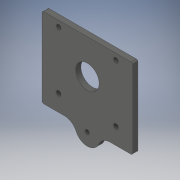
# Autodesk Inventor part: z gearing adapter bottom
Saved by Autodesk Inventor 2019 (Build 230136000, 136)
## iProperties
Created: 2018-07-27
Part Number: z gearing adapter bottom
Material: Generic
Document SubType Name: Modeling
Designer: torba
Density: 1 g/cm^3
Appearance: Gray
Author: torba
Autodesk Inventor part; units mm, degrees
ref_plane "YZ Plane" through (0, 0, 0) normal (1, 0, 0) x (0, 1, 0)
ref_plane "XZ Plane" through (0, 0, 0) normal (0, 1, 0) x (-1, 0, 0)
ref_plane "XY Plane" through (0, 0, 0) normal (0, 0, 1) x (1, 0, 0)
sketch "Sketch1" plane through (0, 0, 0) normal (0, 0, 1) x (1, 0, 0)
  arc A0 (44.2015, -79.5823) -> (38.6015, -79.5823) centre (41.4015, -79.5823) ccw
  arc A1 (38.6015, -85.1823) -> (44.2015, -85.1823) centre (41.4015, -85.1823) ccw
  line L0 (38.6015, -85.1823) -> (38.6015, -79.5823)
  line L1 (44.2015, -79.5823) -> (44.2015, -85.1823)
  arc A2 (39.4335, -50.3778) -> (112.9665, -50.3778) centre (76.2, -50.3778) ccw
  arc A3 (112.9665, -44.7898) -> (39.4335, -44.7898) centre (76.2, -44.7898) ccw
  line L2 (39.4335, -50.3778) -> (39.4335, -44.7898)
  line L3 (112.9665, -44.7898) -> (112.9665, -50.3778)
  line L4 (44.2015, -9.9853) -> (44.2015, -15.5853)
  arc A4 (44.2015, -9.9853) -> (38.6015, -9.9853) centre (41.4015, -9.9853) ccw
  line L5 (38.6015, -15.5853) -> (38.6015, -9.9853)
  arc A5 (38.6015, -15.5853) -> (44.2015, -15.5853) centre (41.4015, -15.5853) ccw
  line L6 (108.1985, -85.1823) -> (108.1985, -79.5823)
  arc A6 (108.1985, -85.1823) -> (113.7985, -85.1823) centre (110.9985, -85.1823) ccw
  line L7 (113.7985, -79.5823) -> (113.7985, -85.1823)
  arc A7 (113.7985, -79.5823) -> (108.1985, -79.5823) centre (110.9985, -79.5823) ccw
  line L8 (108.1985, -15.5853) -> (108.1985, -9.9853)
  arc A8 (113.7985, -9.9853) -> (108.1985, -9.9853) centre (110.9985, -9.9853) ccw
  line L9 (113.7985, -9.9853) -> (113.7985, -15.5853)
  arc A9 (108.1985, -15.5853) -> (113.7985, -15.5853) centre (110.9985, -15.5853) ccw
  circle A10 centre (76.2, -47.5838) radius 1.27
  line L10 (6.35, 0.0014) -> (6.35, -109.7489)
  line L11 (152.4, 0) -> (0, 0)
  line L12 (146.05, 0.0027) -> (146.05, -109.7476)
  line L13 (0, -109.7503) -> (152.4, -109.7503)
  line L14 (21.2, 7.4162) -> (131.2, 7.4162)
  line L15 (131.2, 7.4162) -> (131.2, -102.5838)
  line L16 (131.2, -102.5838) -> (21.2, -102.5838)
  line L17 (21.2, -102.5838) -> (21.2, 7.4162)
  line L18 (21.2, 7.4162) -> (131.2, -102.5838) construction
  line L19 (131.2, 7.4162) -> (21.2, -102.5838) construction
  dimension "d0" = 2.8
  dimension "d1" = 36.7665
  dimension "d2" = 2.54
  dimension "d3" = 90
  dimension "d4" = 90
  dimension "d5" = 90
  dimension "d6" = 90
  dimension "d7" = 109.7503
  dimension "d8" = 32.2515
  dimension "d9" = 33.0835
  dimension "d10" = 101.8485
  dimension "d11" = 139.7
  dimension "d12" = 6.35
  dimension "d13" = 38.6015
  dimension "d14" = 6.35
  dimension "d15" = 0.0027
  dimension "d16" = 37.8515
  dimension "d17" = 109.7476
  dimension "d18" = 9.9853
  dimension "d19" = 69.597
  dimension "d20" = 75.197
  dimension "d21" = 79.5823
  dimension "d22" = 44.7898
  dimension "d23" = 50.3778
  dimension "d24" = 47.5838
  dimension "d25" = 69.85
  dimension "d26" = 9.9853
  dimension "d27" = 79.5823
  dimension "d28" = 0.0014
  dimension "d29" = 109.7489
  dimension "d30" = 146.05
  dimension "d31" = 146.05
  dimension "d32" = 110
  dimension "d33" = 110
  dimension "d34" = 17.4015
  constraints: 40 end point, 24 tangent, 20 point on circle, 11 centre point, 10 parallel, 2 horizontal, 2 midpoint, 1 equal radius, 1 perpendicular, 1 vertical
  measures "d0" radius of A8
  measures "d1" radius of A3
  measures "d2" diameter of A10
  measures "d3" angle of L11 L9
  measures "d4" angle of L11 L8
  measures "d5" angle of L11 L1
  measures "d6" angle of L11 L0
  measures "d7" distance between parallel lines of L11 L13
  measures "d8" distance between parallel lines of L12 L7
  measures "d9" distance between parallel lines of L12 L3
  measures "d10" distance between parallel lines of L12 L4
  measures "d11" distance between parallel lines of L12 L10
  measures "d12" distance from line of L11.start L12
  measures "d13" distance from line of L11.start L9
  measures "d14" distance from line of L13.end L12
  measures "d15" distance from line of L12.start L11
  measures "d16" distance from line of L12.start L8
  measures "d17" distance from line of L12.end L11
  measures "d18" distance from line of L9.start L11
  measures "d19" distance from line of L9.start L1
  measures "d20" distance from line of L9.start L0
  measures "d21" distance from line of L7.start L11
  measures "d22" distance from line of L3.start L11
  measures "d23" distance from line of L3.end L11
  measures "d24" distance from line of A10.centre L11
  measures "d25" distance from line of A10.centre L12
  measures "d26" distance from line of L4.start L11
  measures "d27" distance from line of L1.start L11
  measures "d28" distance from line of L10.start L11
  measures "d29" distance from line of L10.end L11
  measures "d30" distance from line of L11.end L12
  measures "d31" distance from line of L13.start L12
  measures "d32" distance between parallel lines of L15 L17
  measures "d33" distance between parallel lines of L16 L14
  measures "d34" distance from line of L16 A1.centre
extrude "Extrusion1" add sketch "Sketch1" along normal blind 6.35 contours L15 L16 L17 L11 | L11 L17 L14 L15
sketch "Sketch4" plane through (0, 0, 6.35) normal (0, 0, 1) x (1, 0, 0)
  line L0 (112.9665, -44.7898) -> (112.9665, -50.3778) projected
  arc A0 (39.4335, -50.3778) -> (112.9665, -50.3778) centre (76.2, -50.3778) ccw projected
  line L1 (39.4335, -50.3778) -> (39.4335, -44.7898) projected
  arc A1 (112.9665, -44.7898) -> (39.4335, -44.7898) centre (76.2, -44.7898) ccw projected
  arc A2 (38.6015, -15.5853) -> (44.2015, -15.5853) centre (41.4015, -15.5853) ccw projected
  line L2 (38.6015, -15.5853) -> (38.6015, -9.9853) projected
  arc A3 (44.2015, -9.9853) -> (38.6015, -9.9853) centre (41.4015, -9.9853) ccw projected
  line L3 (44.2015, -9.9853) -> (44.2015, -15.5853) projected
  line L4 (44.2015, -79.5823) -> (44.2015, -85.1823) projected
  arc A4 (38.6015, -85.1823) -> (44.2015, -85.1823) centre (41.4015, -85.1823) ccw projected
  line L5 (38.6015, -85.1823) -> (38.6015, -79.5823) projected
  arc A5 (44.2015, -79.5823) -> (38.6015, -79.5823) centre (41.4015, -79.5823) ccw projected
  arc A6 (113.7985, -79.5823) -> (108.1985, -79.5823) centre (110.9985, -79.5823) ccw projected
  line L6 (113.7985, -79.5823) -> (113.7985, -85.1823) projected
  arc A7 (108.1985, -85.1823) -> (113.7985, -85.1823) centre (110.9985, -85.1823) ccw projected
  line L7 (108.1985, -85.1823) -> (108.1985, -79.5823) projected
  arc A8 (113.7985, -9.9853) -> (108.1985, -9.9853) centre (110.9985, -9.9853) ccw projected
  line L8 (113.7985, -9.9853) -> (113.7985, -15.5853) projected
  arc A9 (108.1985, -15.5853) -> (113.7985, -15.5853) centre (110.9985, -15.5853) ccw projected
  line L9 (108.1985, -15.5853) -> (108.1985, -9.9853) projected
  line L10 (21.2, 7.4162) -> (21.2, -102.5838) projected
  line L11 (21.2, -102.5838) -> (131.2, -102.5838) projected
  line L12 (131.2, -102.5838) -> (131.2, 7.4162) projected
  line L13 (76.2, -50.3778) -> (76.2, -44.7898)
  line L14 (76.2, 59.6222) -> (76.2, 65.2102)
  circle A10 centre (76.2, -47.5838) radius 0.5
  circle A11 centre (76.2, 62.4162) radius 0.5
  line L15 (131.2, 7.4162) -> (21.2, 7.4162) projected
  point P0 (0, 0)
  dimension "d72" = 1
  dimension "d73" = 1
  constraints: 4 end point, 2 centre point, 2 midpoint, 2 vertical
  measures "d72" diameter of A10
  measures "d73" diameter of A11
sketch "Sketch11" plane through (0, 0, 6.35) normal (0, 0, 1) x (1, 0, 0)
  line L0 (112.9665, -44.7898) -> (112.9665, -50.3778) projected
  arc A0 (39.4335, -50.3778) -> (112.9665, -50.3778) centre (76.2, -50.3778) ccw projected
  line L1 (39.4335, -50.3778) -> (39.4335, -44.7898) projected
  arc A1 (112.9665, -44.7898) -> (39.4335, -44.7898) centre (76.2, -44.7898) ccw projected
  arc A2 (38.6015, -15.5853) -> (44.2015, -15.5853) centre (41.4015, -15.5853) ccw projected
  line L2 (38.6015, -15.5853) -> (38.6015, -9.9853) projected
  arc A3 (44.2015, -9.9853) -> (38.6015, -9.9853) centre (41.4015, -9.9853) ccw projected
  line L3 (44.2015, -9.9853) -> (44.2015, -15.5853) projected
  line L4 (44.2015, -79.5823) -> (44.2015, -85.1823) projected
  arc A4 (38.6015, -85.1823) -> (44.2015, -85.1823) centre (41.4015, -85.1823) ccw projected
  line L5 (38.6015, -85.1823) -> (38.6015, -79.5823) projected
  arc A5 (44.2015, -79.5823) -> (38.6015, -79.5823) centre (41.4015, -79.5823) ccw projected
  arc A6 (113.7985, -79.5823) -> (108.1985, -79.5823) centre (110.9985, -79.5823) ccw projected
  line L6 (113.7985, -79.5823) -> (113.7985, -85.1823) projected
  arc A7 (108.1985, -85.1823) -> (113.7985, -85.1823) centre (110.9985, -85.1823) ccw projected
  line L7 (108.1985, -85.1823) -> (108.1985, -79.5823) projected
  arc A8 (113.7985, -9.9853) -> (108.1985, -9.9853) centre (110.9985, -9.9853) ccw projected
  line L8 (113.7985, -9.9853) -> (113.7985, -15.5853) projected
  arc A9 (108.1985, -15.5853) -> (113.7985, -15.5853) centre (110.9985, -15.5853) ccw projected
  line L9 (108.1985, -15.5853) -> (108.1985, -9.9853) projected
  line L10 (131.2, 7.4162) -> (21.2, 7.4162) projected
  line L11 (21.2, 7.4162) -> (21.2, -102.5838) projected
  line L12 (21.2, -102.5838) -> (131.2, -102.5838) projected
  line L13 (131.2, -102.5838) -> (131.2, 7.4162) projected
  point P0 (0, 0)
extrude "Extrusion8" add sketch "Sketch11" against normal blind 6.35 contours L0 A0 L1 A1
hole "Hole2" at (76.2, -47.5838, 6.35) direction (0, 0, -1) diameter 28.575 end through all
sketch "Sketch12" plane through (0, 0, 6.35) normal (0, 0, 1) x (1, 0, 0)
  circle A0 centre (76.2, -47.5838) radius 14.2875 projected
  arc A1 (38.6015, -15.5853) -> (44.2015, -15.5853) centre (41.4015, -15.5853) ccw projected
  line L0 (38.6015, -15.5853) -> (38.6015, -9.9853) projected
  arc A2 (44.2015, -9.9853) -> (38.6015, -9.9853) centre (41.4015, -9.9853) ccw projected
  line L1 (44.2015, -9.9853) -> (44.2015, -15.5853) projected
  line L2 (44.2015, -79.5823) -> (44.2015, -85.1823) projected
  arc A3 (38.6015, -85.1823) -> (44.2015, -85.1823) centre (41.4015, -85.1823) ccw projected
  line L3 (38.6015, -85.1823) -> (38.6015, -79.5823) projected
  arc A4 (44.2015, -79.5823) -> (38.6015, -79.5823) centre (41.4015, -79.5823) ccw projected
  arc A5 (113.7985, -79.5823) -> (108.1985, -79.5823) centre (110.9985, -79.5823) ccw projected
  line L4 (113.7985, -79.5823) -> (113.7985, -85.1823) projected
  arc A6 (108.1985, -85.1823) -> (113.7985, -85.1823) centre (110.9985, -85.1823) ccw projected
  line L5 (108.1985, -85.1823) -> (108.1985, -79.5823) projected
  arc A7 (113.7985, -9.9853) -> (108.1985, -9.9853) centre (110.9985, -9.9853) ccw projected
  line L6 (113.7985, -9.9853) -> (113.7985, -15.5853) projected
  arc A8 (108.1985, -15.5853) -> (113.7985, -15.5853) centre (110.9985, -15.5853) ccw projected
  line L7 (108.1985, -15.5853) -> (108.1985, -9.9853) projected
  line L8 (131.2, 7.4162) -> (21.2, 7.4162) projected
  line L9 (21.2, 7.4162) -> (21.2, -102.5838) projected
  line L10 (21.2, -102.5838) -> (131.2, -102.5838) projected
  line L11 (131.2, -102.5838) -> (131.2, 7.4162) projected
  line L12 (21.2, -102.5838) -> (21.2, 7.4162) projected
  line L13 (131.2, 7.4162) -> (131.2, -102.5838) projected
  line L14 (21.2, 7.4162) -> (131.2, 7.4162)
  line L15 (131.2, 7.4162) -> (131.2, 0.8147)
  line L16 (131.2, 0.8147) -> (21.2, 0.8147)
  line L17 (21.2, 0.8147) -> (21.2, 7.4162)
  point P0 (0, 0)
  dimension "d103" = 8
  constraints: 8 end point, 2 parallel, 1 horizontal, 1 perpendicular, 1 point on line
  measures "d103" distance edge to line of A2 L16
extrude "Extrusion9" cut sketch "Sketch12" against normal blind 6.35 contours L11 L16 L9 L8
sketch "Sketch13" plane through (0, 0, 6.35) normal (0, 0, 1) x (1, 0, 0)
  line L0 (131.2, 0.8147) -> (21.2, 0.8147) projected
  line L1 (21.2, 0.8147) -> (21.2, -102.5838) projected
  line L2 (21.2, -102.5838) -> (131.2, -102.5838) projected
  line L3 (131.2, -102.5838) -> (131.2, 0.8147) projected
  arc A0 (113.7985, -9.9853) -> (108.1985, -9.9853) centre (110.9985, -9.9853) ccw projected
  line L4 (113.7985, -9.9853) -> (113.7985, -15.5853) projected
  arc A1 (108.1985, -15.5853) -> (113.7985, -15.5853) centre (110.9985, -15.5853) ccw projected
  line L5 (108.1985, -15.5853) -> (108.1985, -9.9853) projected
  arc A2 (113.7985, -79.5823) -> (108.1985, -79.5823) centre (110.9985, -79.5823) ccw projected
  line L6 (113.7985, -79.5823) -> (113.7985, -85.1823) projected
  arc A3 (108.1985, -85.1823) -> (113.7985, -85.1823) centre (110.9985, -85.1823) ccw projected
  line L7 (108.1985, -85.1823) -> (108.1985, -79.5823) projected
  line L8 (44.2015, -79.5823) -> (44.2015, -85.1823) projected
  arc A4 (38.6015, -85.1823) -> (44.2015, -85.1823) centre (41.4015, -85.1823) ccw projected
  line L9 (38.6015, -85.1823) -> (38.6015, -79.5823) projected
  arc A5 (44.2015, -79.5823) -> (38.6015, -79.5823) centre (41.4015, -79.5823) ccw projected
  arc A6 (38.6015, -15.5853) -> (44.2015, -15.5853) centre (41.4015, -15.5853) ccw projected
  line L10 (38.6015, -15.5853) -> (38.6015, -9.9853) projected
  arc A7 (44.2015, -9.9853) -> (38.6015, -9.9853) centre (41.4015, -9.9853) ccw projected
  line L11 (44.2015, -9.9853) -> (44.2015, -15.5853) projected
  circle A8 centre (76.2, -47.5838) radius 14.2875 projected
  line L12 (41.4015, -85.1823) -> (41.4015, -79.5823)
  line L13 (41.4015, -15.5853) -> (41.4015, -9.9853)
  line L14 (110.9985, -85.1823) -> (110.9985, -79.5823)
  line L15 (41.4015, -85.1823) -> (41.4015, -79.5823) construction
  line L16 (44.2015, -85.1823) -> (44.2015, -79.5823)
  line L17 (38.6015, -79.5823) -> (38.6015, -85.1823)
  arc A9 (38.6015, -85.1823) -> (44.2015, -85.1823) centre (41.4015, -85.1823) ccw
  arc A10 (44.2015, -79.5823) -> (38.6015, -79.5823) centre (41.4015, -79.5823) ccw
  arc A11 (44.2015, -9.9853) -> (38.6015, -9.9853) centre (41.4015, -9.9853) ccw projected
  line L18 (41.4015, -15.5853) -> (41.4015, -9.9853) construction
  line L19 (44.2015, -15.5853) -> (44.2015, -9.9853)
  line L20 (38.6015, -9.9853) -> (38.6015, -15.5853)
  arc A12 (38.6015, -15.5853) -> (44.2015, -15.5853) centre (41.4015, -15.5853) ccw
  arc A13 (44.2015, -9.9853) -> (38.6015, -9.9853) centre (41.4015, -9.9853) ccw
  line L21 (110.9985, -85.1823) -> (110.9985, -79.5823) construction
  line L22 (113.7985, -85.1823) -> (113.7985, -79.5823)
  line L23 (108.1985, -79.5823) -> (108.1985, -85.1823)
  arc A14 (108.1985, -85.1823) -> (113.7985, -85.1823) centre (110.9985, -85.1823) ccw
  arc A15 (113.7985, -79.5823) -> (108.1985, -79.5823) centre (110.9985, -79.5823) ccw
  line L24 (110.9985, -15.5853) -> (110.9985, -9.9853) construction
  line L25 (113.7985, -15.5853) -> (113.7985, -9.9853)
  line L26 (108.1985, -9.9853) -> (108.1985, -15.5853)
  arc A16 (108.1985, -15.5853) -> (113.7985, -15.5853) centre (110.9985, -15.5853) ccw
  arc A17 (113.7985, -9.9853) -> (108.1985, -9.9853) centre (110.9985, -9.9853) ccw
  line L27 (110.9985, -9.9853) -> (110.9985, -15.5853)
  circle A18 centre (110.9985, -12.7853) radius 2.8
  circle A19 centre (41.4015, -12.7853) radius 2.8
  circle A20 centre (41.4015, -82.3823) radius 2.8
  circle A21 centre (110.9985, -82.3823) radius 2.8
  point P0 (0, 0)
  dimension "d108" = 2.8
  dimension "d109" = 2.8
  dimension "d110" = 2.8
  constraints: 40 end point, 21 tangent, 16 point on circle, 12 centre point, 8 equal length, 4 coincident, 4 midpoint, 3 vertical
  measures "d108" radius of A17
  measures "d109" radius of A15
  measures "d110" radius of A10
extrude "Extrusion10" add sketch "Sketch13" against normal blind 6.35 contours L4 A18 L5 A0 | L4 A1 L5 A18 | L6 A21 L7 A2 | L6 A3 L7 A21 | L8 A20 L9 A5 | L8 A4 L9 A20 | L10 A19 L11 A6 | L10 A7 L11 A19
sketch "Sketch17" plane through (0, 0, 6.35) normal (0, 0, 1) x (1, 0, 0)
  circle A0 centre (76.2, -105.7258) radius 4
  circle A1 centre (76.2, -105.7258) radius 2.5
  circle A2 centre (41.4015, -82.3823) radius 2.8
  circle A3 centre (41.4015, -82.3823) radius 2.8 projected
  circle A4 centre (76.2, -105.7258) radius 15
  line L0 (21.2, -102.5838) -> (131.2, -102.5838) projected
  line L1 (131.2, -102.5838) -> (131.2, 0.8147) projected
  line L2 (131.2, 0.8147) -> (21.2, 0.8147) projected
  line L3 (21.2, 0.8147) -> (21.2, -102.5838) projected
  circle A5 centre (110.9985, -12.7853) radius 2.8 projected
  circle A6 centre (110.9985, -82.3823) radius 2.8 projected
  circle A7 centre (41.4015, -82.3823) radius 2.8 projected
  circle A8 centre (41.4015, -12.7853) radius 2.8 projected
  circle A9 centre (76.2, -47.5838) radius 14.2875 projected
  dimension "d117" = 30
  dimension "d118" = 8
  dimension "d119" = 5
  dimension "d120" = 5.6
  dimension "d121" = 41.9029
  dimension "d122" = 0
  dimension "d123" = 55
  constraints: 4 centre point, 1 coincident, 1 concentric
  measures "d117" diameter of A4
  measures "d118" diameter of A0
  measures "d119" diameter of A1
  measures "d120" diameter of A2
  measures "d121" distance of A3.centre A4.centre
  measures "d122" distance of A3.centre A2.centre
  measures "d123" distance from line of A0.centre L1
extrude "Extrusion12" add sketch "Sketch17" against normal blind 6.35 contours A0 L0 | A0 L0 A4 | L0 A0 | A0 L0 A4
fillet "Fillet4" radius 15 2 edges at (90.8672, -102.5838, 3.175) (61.5328, -102.5838, 3.175)
sketch "Sketch19" plane through (21.2, 0.8147, 6.35) normal (0, 1, 0) x (1, 0, 0)
  line L0 (110, 0) -> (0, 0) projected
  line L1 (110, 6.35) -> (110, 0) projected
  line L2 (0, 6.35) -> (110, 6.35) projected
  line L3 (0, 0) -> (0, 6.35) projected
  point P0 (-21.2, 6.35)
extrude "Extrusion13" cut sketch "Sketch19" against normal blind 6.35
fillet "Fillet5" radius 2 4 edges at (131.2, -5.5353, 3.175) (131.2, -102.5838, 3.175) (21.2, -102.5838, 3.175) (21.2, -5.5353, 3.175)
sketch "Sketch15" plane through (0, 0, 6.35) normal (0, 0, 1) x (1, 0, 0)
  circle A0 centre (110.9985, -12.7853) radius 2.8 projected
  circle A1 centre (110.9985, -82.3823) radius 2.8 projected
  line L0 (131.2, 0.8147) -> (21.2, 0.8147) projected
  line L1 (21.2, 0.8147) -> (21.2, -102.5838) projected
  line L2 (21.2, -102.5838) -> (131.2, -102.5838) projected
  line L3 (131.2, -102.5838) -> (131.2, 0.8147) projected
  circle A2 centre (41.4015, -82.3823) radius 2.8 projected
  circle A3 centre (41.4015, -12.7853) radius 2.8 projected
  circle A4 centre (76.2, -47.5838) radius 14.2875 projected
  circle A5 centre (41.4015, -82.3823) radius 3.75
  circle A6 centre (110.9985, -82.3823) radius 3.75
  point P0 (0, 0)
  dimension "d111" = 7.5
  dimension "d112" = 7.5
  constraints: 2 centre point, 2 coincident
  measures "d111" diameter of A5
  measures "d112" diameter of A6
body "Solid1"
